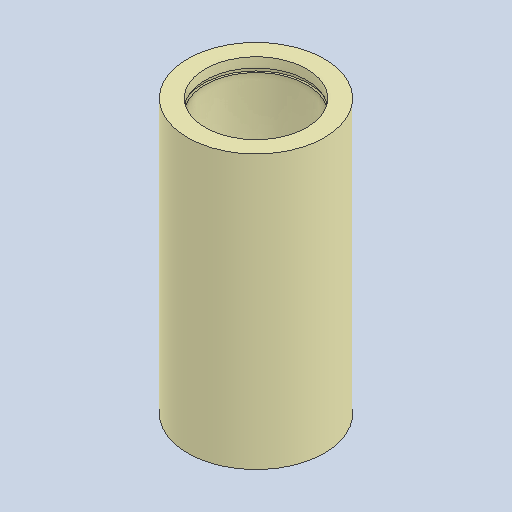
# Autodesk Inventor part: корпус
Saved by Autodesk Inventor 2023.2 (Build 272271030, 271C)
## iProperties
Created: 2024-02-27
Part Number: корпус
Material: Типовые
Document SubType Name: Modeling
Designer: user
Density: 1 g/cm^3
Appearance: По умолчанию
Author: user
Autodesk Inventor part; units mm, degrees
ref_plane "YZ Plane" through (0, 0, 0) normal (1, 0, 0) x (0, 1, 0)
ref_plane "XZ Plane" through (0, 0, 0) normal (0, 1, 0) x (-1, 0, 0)
ref_plane "XY Plane" through (0, 0, 0) normal (0, 0, 1) x (1, 0, 0)
sketch "Эскиз1" plane through (0, 0, 0) normal (0, 0, 1) x (1, 0, 0)
  line L0 (0, 0) -> (0, -140)
  line L1 (0, 0) -> (26, 0) construction
  line L2 (35, 0) -> (35, -140)
  line L3 (35, -140) -> (26, -140)
  line L4 (26, 0) -> (26, -5)
  line L5 (26, -5) -> (27, -5)
  line L6 (27, -5) -> (27, -7)
  line L7 (27, -7) -> (26, -7)
  line L8 (26, -7) -> (26, -123)
  line L9 (26, -123) -> (27, -123)
  line L10 (27, -123) -> (27, -125)
  line L11 (27, -125) -> (26, -125)
  line L12 (26, -125) -> (26, -140)
  line L13 (26, -140) -> (0, -140) construction
  line L14 (26, 0) -> (35, 0)
  point P0 (26, -7)
  point P1 (28.5, 0)
  dimension "d0" = 140
  dimension "d1" = 70
  dimension "d3" = 54
  dimension "d4" = 52
  dimension "d5" = 2
  dimension "d6" = 2
  dimension "d13" = 5
  dimension "d14" = 15
  constraints: 30 end point, 10 perpendicular, 4 point on line, 3 horizontal, 2 collinear, 2 vertical
  measures "d0" distance of L0.start L0.end
  measures "d1" diameter of L2 L0
  measures "d3" diameter of L6 L0
  measures "d4" diameter of L4 L0
  measures "d5" distance of L5.end L6.end
  measures "d6" distance of L9.end L10.end
  measures "d13" distance between parallel lines of L5 L14
  measures "d14" distance between parallel lines of L3 L11
revolve "Вращение1" add sketch "Эскиз1" angle 360 about axis through (0, 0, 0) along (0, -1, 0)
equation "\"d14\" = my_parameter"
equation "\"my_parameter\" = 15"
